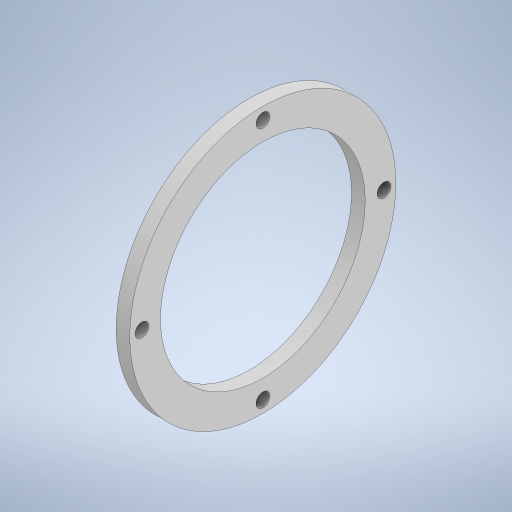
# Autodesk Inventor part: base_bearing_holder
Saved by Autodesk Inventor 2024 (Build 280153000, 153)
## iProperties
Created: 2025-12-08
Part Number: base_bearing_holder
Material: Generic
Document SubType Name: Modeling
Designer: schar
Density: 1 g/cm^3
Appearance: Default
Author: schar
Autodesk Inventor part; units mm, degrees
ref_plane "YZ Plane" through (0, 0, 0) normal (1, 0, 0) x (0, 1, 0)
ref_plane "XZ Plane" through (0, 0, 0) normal (0, 1, 0) x (-1, 0, 0)
ref_plane "XY Plane" through (0, 0, 0) normal (0, 0, 1) x (1, 0, 0)
sketch "Sketch1" plane through (0, 0, 0) normal (1, 0, 0) x (0, 1, 0)
  circle A0 centre (0, 0) radius 16
  circle A1 centre (0, 0) radius 19.5
  dimension "d0" = 32
  dimension "d1" = 39
  constraints: 2 centre point, 2 coincident
  measures "d0" diameter of A0
  measures "d1" diameter of A1
extrude "Extrusion1" add sketch "Sketch1" along normal blind 2 and the other way blind 2 contours A0
sketch "Sketch2" plane through (2, 0, 0) normal (1, 0, 0) x (0, 0, -1)
  circle A0 centre (0, 0) radius 19.5
  circle A1 centre (0, 0) radius 16
  dimension "d6" = 39
  constraints: 2 centre point, 2 coincident
  measures "d6" diameter of A0
extrude "Extrusion2" add sketch "Sketch2" against normal blind 2
sketch "Sketch3" plane through (-2, 0, 0) normal (-1, 0, 0) x (0, 0, 1)
  circle A0 centre (0, 0) radius 16
  circle A1 centre (0, 0) radius 15
  dimension "d9" = 30
  constraints: 2 centre point, 2 coincident
  measures "d9" diameter of A1
extrude "Extrusion3" cut sketch "Sketch3" against normal blind 10 contours A1
sketch "Sketch5" plane through (0, 0, 0) normal (-1, 0, 0) x (0, 0, 1)
  circle A0 centre (0, 0) radius 17.75
  circle A1 centre (0, 17.75) radius 1
  circle A2 centre (-17.75, 0) radius 1
  circle A3 centre (0, -17.75) radius 1
  circle A4 centre (17.75, 0) radius 1
  dimension "d12" = 35.5
  dimension "d13" = 2
  dimension "d16" = 360
  constraints: 4 centre point, 1 coincident, 1 vertical alignment, 11 other
  measures "d13" diameter of A1
hole "Hole1" at (0, 17.75, 0) at (0, 0, 17.75) at (0, -17.75, 0) at (0, 0, -17.75) direction (1, 0, 0) diameter 2 end through all
sketch "Sketch7" plane through (-2, 0, 0) normal (-1, 0, 0) x (0, 0, 1)
  circle A0 centre (0, 0) radius 15
  circle A1 centre (0, 0) radius 16
  constraints: 2 centre point, 2 coincident
extrude "Extrusion4" cut sketch "Sketch7" against normal blind 2
body "Solid1"
